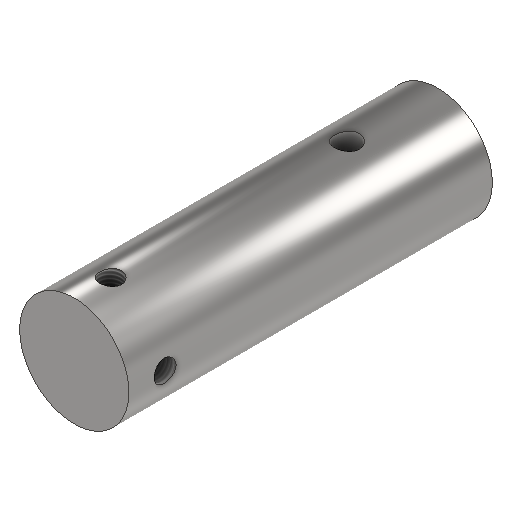
# Autodesk Inventor part: rotary_transfer_shaft_5
Saved by Autodesk Inventor 2026.2 (Build 302298000, 298)
## iProperties
Created: 2026-05-26
Part Number: rotary_transfer_shaft_5
Material: ステンレス鋼
Document SubType Name: Modeling
Designer: zetsu
Density: 8 g/cm^3
Appearance: 半つや出し
Author: zetsu
Autodesk Inventor part; units mm, degrees
sketch "スケッチ1" plane through (0, 0, 0) normal (0, 0, 1) x (1, 0, 0)
  circle A0 centre (0, 0) radius 7.5
  dimension "d0" = 15
  constraints: 1 centre point, 1 coincident
  measures "d0" diameter of A0
extrude "押し出し1" add sketch "スケッチ1" along normal blind 50
sketch "スケッチ2" plane through (0, 0, 0) normal (0, 0, -1) x (-1, 0, 0)
  arc A0 (-2.9394, 3) -> (2.9394, 3) centre (0, 0) ccw
  line L0 (-2.9394, 3) -> (2.9394, 3)
  point P0 (-3.1305, 2.8)
  dimension "d3" = 4.2
  dimension "d4" = 3
  constraints: 3 point on circle, 2 end point, 1 centre point, 1 coincident, 1 horizontal
  measures "d3" radius of A0
  measures "d4" vertical distance of point (0, 0) L0.start
extrude "押し出し2" cut sketch "スケッチ2" against normal blind 30
ref_plane "作業平面1" through (7.5, 0, 0) normal (1, 0, 0) x (0, 1, 0)
ref_plane "作業平面2" through (-7.5, 0, 0) normal (1, 0, 0) x (0, 1, 0)
ref_plane "作業平面3" through (0, 7.5, 0) normal (0, 1, 0) x (-1, 0, 0)
ref_plane "作業平面4" through (0, -7.5, 0) normal (0, 1, 0) x (-1, 0, 0)
sketch "スケッチ3" plane through (7.5, 0, 0) normal (1, 0, 0) x (0, 1, 0)
  circle A0 centre (0, 45) radius 1.5
  line L0 (7.5, 50) -> (-7.5, 50) projected
  point P0 (0, 0)
  dimension "d11" = 3
  dimension "d12" = 5
  constraints: 1 centre point
  measures "d11" diameter of A0
  measures "d12" distance from line of A0.centre L0
sketch "スケッチ4" plane through (-7.5, 0, 0) normal (1, 0, 0) x (0, 1, 0)
  circle A0 centre (0, 45) radius 1.5
  line L0 (7.5, 50) -> (-7.5, 50) projected
  point P0 (0, 0)
  dimension "d13" = 3
  dimension "d14" = 5
  constraints: 1 centre point
  measures "d13" diameter of A0
  measures "d14" distance from line of L0 A0.centre
extrude "押し出し3" cut sketch "スケッチ3" against normal blind 5
extrude "押し出し4" cut sketch "スケッチ4" along normal blind 5
sketch "スケッチ5" plane through (0, 7.5, 0) normal (0, 1, 0) x (-1, 0, 0)
  circle A0 centre (0, 45) radius 1.5
  line L0 (7.5, 50) -> (-7.5, 50) projected
  point P0 (0, 0)
  dimension "d19" = 3
  dimension "d20" = 5
  constraints: 1 centre point
  measures "d19" diameter of A0
  measures "d20" distance from line of L0 A0.centre
sketch "スケッチ6" plane through (0, -7.5, 0) normal (0, 1, 0) x (-1, 0, 0)
  circle A0 centre (0, 45) radius 1.5
  line L0 (7.5, 50) -> (-7.5, 50) projected
  point P0 (0, 0)
  dimension "d21" = 3
  dimension "d22" = 5
  constraints: 1 centre point
  measures "d21" diameter of A0
  measures "d22" distance from line of L0 A0.centre
extrude "押し出し5" cut sketch "スケッチ5" against normal blind 5
extrude "押し出し6" cut sketch "スケッチ6" along normal blind 5
thread "ねじ1" size "M3x0.5" class "6H" standard "ANSI Metric M Profile" full length
thread "ねじ2" size "M3x0.5" class "6H" standard "ANSI Metric M Profile" full length
thread "ねじ3" size "M3x0.5" class "6H" standard "ANSI Metric M Profile" full length
thread "ねじ4" size "M3x0.5" class "6H" standard "ANSI Metric M Profile" full length
sketch "スケッチ7" plane through (0, 7.5, 0) normal (0, 1, 0) x (-1, 0, 0)
  circle A0 centre (0, 12.5) radius 1.7
  point P0 (0, 0)
  dimension "d35" = 3.4
  dimension "d36" = 12.5
  constraints: 1 centre point
  measures "d35" diameter of A0
  measures "d36" distance of point (0, 0) A0.centre
extrude "押し出し7" cut sketch "スケッチ7" against normal through all
